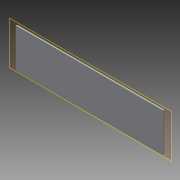
# Autodesk Inventor part: Panel_back
Saved by Autodesk Inventor 2013 (Build 170138000, 138)
## iProperties
Created: 2013-02-02
Part Number: Panel_back
Material: Aluminum 6061
Document SubType Name: Modeling
Designer: xylzlyx
Density: 1 g/cm^3
Author: xylzlyx
Autodesk Inventor part; units mm, degrees
ref_plane "YZ Plane" through (0, 0, 0) normal (1, 0, 0) x (0, 1, 0)
ref_plane "XZ Plane" through (0, 0, 0) normal (0, 1, 0) x (-1, 0, 0)
ref_plane "XY Plane" through (0, 0, 0) normal (0, 0, 1) x (1, 0, 0)
ref_plane "Work Plane1" through (0, 0, -12.7) normal (0, 0, 1) x (1, 0, 0)
sketch "Sketch1" plane through (0, 0, -12.7) normal (0, 0, 1) x (1, 0, 0)
  line L0 (0, -104.216) -> (0, -100.9921) construction
  line L1 (0, -100.9921) -> (381, -100.9921) construction
  line L2 (381, -100.9921) -> (381, -104.216) construction
  line L3 (381, -104.216) -> (0, -104.216) construction
  line L4 (381, 3.175) -> (381, 0) construction
  line L5 (381, 0) -> (0, 0) construction
  line L6 (0, 0) -> (0, 3.175) construction
  line L7 (0, 3.175) -> (381, 3.175) construction
  line L8 (381, -100.9921) -> (0, -100.9921)
  line L9 (0, -100.9921) -> (0, 0)
  line L10 (0, 0) -> (381, 0)
  line L11 (381, 0) -> (381, -100.9921)
  constraints: 24 end point, 5 horizontal, 4 coincident, 4 vertical, 2 parallel, 1 perpendicular, 7 other
extrude "BackPanel" add sketch "Sketch1" along normal blind 3.175
fillet "Fillet1" radius 1 4 edges at (381, -100.9921, -11.1125) (381, 0, -11.1125) (0, 0, -11.1125) (0, -100.9921, -11.1125)
body "Solid1"
